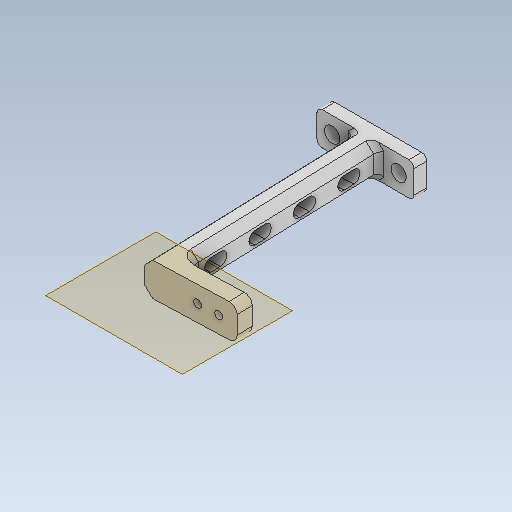
# Autodesk Inventor part: 2200_support_3
Saved by Autodesk Inventor 2020 (Build 240168000, 168)
## iProperties
Created: 2019-10-23
Part Number: 2200_support_3
Material: Generic
Document SubType Name: Modeling
Designer: psrob
Density: 1 g/cm^3
Appearance: Default
Author: psrob
Autodesk Inventor part; units mm, degrees
ref_plane "YZ Plane" through (0, 0, 0) normal (1, 0, 0) x (0, 1, 0)
ref_plane "XZ Plane" through (0, 0, 0) normal (0, 1, 0) x (-1, 0, 0)
ref_plane "Work Plane1" through (13.385568, -75.691032, 8.789403) normal (0, 1, 0) x (-1, 0, 0)
sketch "Sketch1" plane through (13.385568, -75.691032, 8.789403) normal (0, 1, 0) x (-1, 0, 0)
  line L0 (-15.308723, 11.625075) -> (21.189984, 11.849305)
  arc A0 (24.208358, 8.867791) -> (21.189984, 11.849305) centre (21.208414, 8.849361) ccw
  line L1 (24.208358, 8.867791) -> (24.271339, -1.383926)
  arc A1 (21.289826, -4.402299) -> (24.271339, -1.383926) centre (21.271396, -1.402356) ccw
  line L2 (21.289826, -4.402299) -> (-15.101084, -4.625866)
  arc A2 (-15.101084, -4.625866) -> (-19.184317, -8.625) centre (-15.184317, -8.625) ccw
  line L3 (-19.184317, -8.625) -> (-19.184317, -17.625)
  arc A3 (-19.184317, -17.625) -> (-17.184317, -19.625) centre (-17.184317, -17.625) ccw
  line L4 (-17.184317, -19.625) -> (-13.184317, -19.625)
  arc A4 (-13.184317, -19.625) -> (-11.184317, -17.625) centre (-13.184317, -17.625) ccw
  line L5 (-11.184317, -17.625) -> (-11.184317, -14.429635)
  arc A5 (-9.250498, -12.430731) -> (-11.184317, -14.429635) centre (-9.184317, -14.429635) ccw
  line L6 (-9.250498, -12.430731) -> (26.41284, -11.249964)
  arc A6 (26.41284, -11.249964) -> (29.313512, -8.233177) centre (26.313568, -8.251607) ccw
  line L7 (29.313512, -8.233177) -> (29.168899, 15.305992)
  arc A7 (29.168899, 15.305992) -> (26.265471, 18.286008) centre (26.168956, 15.287561) ccw
  line L8 (26.265471, 18.286008) -> (-15.076057, 19.61672)
  arc A8 (-15.076057, 19.61672) -> (-15.308723, 11.625075) centre (-15.333297, 15.625) ccw
  circle A9 centre (-15.184317, -8.625) radius 1.5
  circle A10 centre (-15.333297, 15.625) radius 1.5
  circle A11 centre (-15.184317, -15.625) radius 1.5
  line L9 (-9.250498, -12.430731) -> (25.730334, -11.272561)
  line L10 (90.666703, -101.625) -> (-109.333297, -101.625)
  line L11 (25.730334, -11.272561) -> (28.721786, -101.625)
  line L12 (28.721786, -101.625) -> (18.721786, -101.625)
  line L13 (18.721786, -101.625) -> (16.00836, -19.669907)
  line L14 (16.00836, -19.669907) -> (-8.977949, -20.497171)
  line L15 (-9.250498, -12.430731) -> (-8.977949, -20.497171)
  point P0 (13.385568, -8.789403)
  dimension "d0" = 35
  dimension "d1" = 10
  dimension "d2" = 82
  dimension "d3" = 25
  constraints: 12 end point, 3 point on line, 2 parallel, 1 perpendicular
  measures "d0" distance of L6.start L9.end
  measures "d1" distance of L11.end L12.end
  measures "d2" distance of L12.end L13.end
  measures "d3" distance of L13.end L14.end
ref_plane "Work Plane2" through (-15.928, -88.691032, -10.835597) normal (0, -1, 0) x (1, 0, 0)
extrude "Extrusion1" add sketch "Sketch1" against normal up to surface (13 mm away) contours L11 L10 L13 L14 L15 L6
sketch "Sketch2" plane through (-2.622791, -88.691032, -10.880503) normal (-0.0330906, 0, -0.9994524) x (-0.9994524, 0, 0.0330906)
  circle A0 centre (-18.005476, 6.5) radius 1.5
  circle A1 centre (-10.005476, 6.5) radius 1.5
  point P0 (-2.261313, 88.691032)
extrude "Extrusion2" cut sketch "Sketch2" against normal blind 10
sketch "Sketch3" plane through (13.385568, -75.691032, 8.789403) normal (0, 1, 0) x (1, 0, 0)
  line L0 (109.333297, 100.625) -> (-90.666703, 100.625)
  line L1 (8.977949, 20.497171) -> (-16.00836, 19.669907)
  line L2 (-16.00836, 19.669907) -> (-18.721786, 101.625)
  line L3 (-18.721786, 101.625) -> (-28.721786, 101.625)
  line L4 (-28.721786, 101.625) -> (-25.730334, 11.272561)
  line L5 (-25.730334, 11.272561) -> (9.250498, 12.430731)
  line L6 (9.250498, 12.430731) -> (8.977949, 20.497171)
  point P0 (-13.385568, 8.789403)
  point P1 (-28.688677, 100.625)
  point P2 (-18.688677, 100.625)
extrude "Extrusion3" cut sketch "Sketch3" against normal blind 18 contours L0 L4 L3 L2
sketch "Sketch4" plane through (13.385568, -75.691032, 8.789403) normal (0, 1, 0) x (1, 0, 0)
  line L0 (-18.688677, 100.625) -> (-28.688677, 100.625)
  line L1 (-28.688677, 100.625) -> (-25.730334, 11.272561)
  line L2 (-25.730334, 11.272561) -> (9.250498, 12.430731)
  line L3 (9.250498, 12.430731) -> (8.977949, 20.497171)
  line L4 (8.977949, 20.497171) -> (-16.00836, 19.669907)
  line L5 (-16.00836, 19.669907) -> (-18.688677, 100.625)
  line L6 (109.333297, 100.625) -> (-90.666703, 100.625)
  line L7 (-28.688677, 100.625) -> (-42.688677, 100.625)
  line L8 (-18.688677, 100.625) -> (-28.688677, 100.625)
  line L9 (-18.688677, 100.625) -> (-4.688677, 100.625)
  line L10 (-4.688677, 100.625) -> (-4.688677, 95.625)
  line L11 (-4.688677, 95.625) -> (-18.523134, 95.625)
  line L12 (-28.523134, 95.625) -> (-42.688677, 95.625)
  line L13 (-42.688677, 95.625) -> (-42.688677, 100.625)
  point P0 (-13.385568, 8.789403)
  dimension "d10" = 14
  dimension "d11" = 14
  dimension "d12" = 5
  constraints: 12 end point, 6 point on line, 2 perpendicular, 1 vertical
  measures "d10" distance of L0.end L7.end
  measures "d11" distance of L0.start L9.end
  measures "d12" distance of L9.end L10.end
extrude "Extrusion4" add sketch "Sketch4" against normal up to surface (13 mm away) contours L6 L10 L11 L5 | L1 L12 L13 L6
sketch "Sketch5" plane through (-5.137565, -75.691032, -86.835597) normal (0, 0, 1) x (1, 0, 0)
  line L0 (-24.165543, -13) -> (-10, -13)
  line L1 (-10, 0) -> (-10, -13)
  line L2 (-24.165543, 0) -> (-10, 0)
  line L3 (-24.165543, 0) -> (-24.165543, -13)
  line L4 (0, -13) -> (13.834457, -13)
  line L5 (13.834457, 0) -> (13.834457, -13)
  line L6 (0, 0) -> (13.834457, 0)
  line L7 (0, -13) -> (0, 0)
  line L8 (-24.165543, -6.5) -> (-18.165543, -6.5)
  circle A0 centre (-18.165543, -6.5) radius 3
  line L9 (13.834457, -6.5) -> (7.834457, -6.5)
  circle A1 centre (7.834457, -6.5) radius 3
  point P0 (5.137565, 75.691032)
  dimension "d15" = 6
  dimension "d16" = 6
  dimension "d17" = 6
  dimension "d18" = 6
  constraints: 4 end point, 2 centre point, 2 coincident, 2 horizontal, 2 midpoint
  measures "d15" distance of L8.start L8.end
  measures "d16" diameter of A0
  measures "d17" distance of L9.start L9.end
  measures "d18" diameter of A1
extrude "Extrusion5" cut sketch "Sketch5" against normal blind 18 contours A0 | A1
thicken "Thicken1" operation add thickness 2 both sides no extend neighbours yes toward (0.0330906, 0, 0.9994524) faces at (9.099546, -77.361344, -11.268615)
chamfer "Chamfer1" distance 3 angle 45 4 edges at (-3.8471, -88.691, -47.8586) (-13.7412, -88.691, -44.6594) (-3.8471, -75.691, -47.8586) (-13.7412, -75.691, -44.6594)
fillet "Fillet1" radius 2 6 edges at (-13.6367, -77.191, -86.8356) (-15.1376, -82.191, -86.8356) (-13.6367, -87.191, -86.8356) (-6.6384, -77.191, -86.8356) (-5.1376, -82.191, -86.8356) (-6.6384, -87.191, -86.8356)
fillet "Fillet2" radius 2 4 edges at (8.6969, -75.691, -89.3356) (8.6969, -88.691, -89.3356) (-29.3031, -75.691, -89.3356) (-29.3031, -88.691, -89.3356)
fillet "Fillet3" radius 5 3 edges at (-4.0558, -87.191, -8.832) (-2.5566, -82.191, -8.8816) (-4.0558, -77.191, -8.832)
fillet "Fillet4" radius 3 2 edges at (22.5336, -88.691, -6.6751) (22.5336, -75.691, -6.6751)
sketch "Sketch6" plane through (-12.344766, -85.691032, -2.483158) normal (-0.9994524, 0, 0.0330906) x (0.0330906, 0, 0.9994524)
  line L0 (-82.463781, -0.000133) -> (-82.463781, 7.000133)
  ellipse E0 centre (-82.397564, -2.828427) end of major axis (-82.491183, -0.000774) minor radius 2 (-82.444386, 0) -> (-82.463781, -0.000133) ccw
  line L1 (0, 0) -> (-82.444386, 0)
  line L2 (0, 7) -> (0, 0)
  line L3 (-82.444386, 7) -> (0, 7)
  ellipse E1 centre (-82.397564, 9.828427) end of major axis (-82.491183, 7.000774) minor radius 2 (-82.463781, 7.000133) -> (-82.444386, 7) ccw
  line L4 (0, 7) -> (0, 0)
  line L5 (0, 3.5) -> (-18, 3.5)
  line L6 (-16, 3.5) -> (-20, 3.5) construction
  line L7 (-16, 6) -> (-20, 6)
  line L8 (-20, 1) -> (-16, 1)
  arc A0 (-16, 1) -> (-16, 6) centre (-16, 3.5) ccw
  arc A1 (-20, 6) -> (-20, 1) centre (-20, 3.5) ccw
  arc A2 (-38, 6) -> (-38, 1) centre (-38, 3.5) ccw
  line L9 (-34, 6) -> (-38, 6)
  line L10 (-38, 1) -> (-34, 1)
  arc A3 (-34, 1) -> (-34, 6) centre (-34, 3.5) ccw
  arc A4 (-56, 6) -> (-56, 1) centre (-56, 3.5) ccw
  line L11 (-52, 6) -> (-56, 6)
  line L12 (-56, 1) -> (-52, 1)
  arc A5 (-52, 1) -> (-52, 6) centre (-52, 3.5) ccw
  arc A6 (-74, 6) -> (-74, 1) centre (-74, 3.5) ccw
  line L13 (-70, 6) -> (-74, 6)
  line L14 (-74, 1) -> (-70, 1)
  arc A7 (-70, 1) -> (-70, 6) centre (-70, 3.5) ccw
  point P0 (2.890293, 85.691032)
  dimension "d30" = 18
  dimension "d31" = 2
  dimension "d32" = 5
  dimension "d35" = 18
  constraints: 22 end point, 16 point on circle, 8 centre point, 4 tangent, 3 horizontal, 2 midpoint, 1 parallel, 32 other
  measures "d30" distance of L5.start L5.end
  measures "d31" distance of L5.end L6.end
  measures "d32" diameter of A1
  measures "d35" distance of L6.end A2.centre
extrude "Extrusion6" cut sketch "Sketch6" against normal blind 18 contours A0 L8 A1 L7 | L9 A3 L10 A2 | L11 A5 L12 A4 | L13 A7 L14 A6
body "Solid1"
